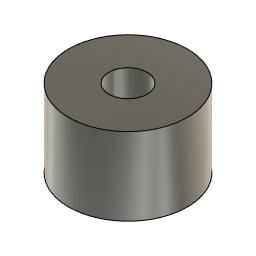
Water_Gun_Stand (Autodesk Fusion 360 archive; units mm, degrees)
design "c-clamp_base_v.1.0.0.0"
Autodesk Fusion 360 part; units mm, degrees
sketch "Base" plane through (0, 0, 0) normal (0, 0, 1) x (1, 0, 0)
  circle A0 centre (0, 0) radius 13
  circle A1 centre (24.2, 0) radius 11.2
  line L0 (25.0331, 11.169) -> (0.9669, 12.964)
  line L1 (0.9669, -12.964) -> (25.0331, -11.169)
  line L2 (0, 0) -> (24.2, 0) construction
  circle A2 centre (24.2, 0) radius 8
  line L3 (9.2469, 9.1375) -> (24.795, 7.9778)
  line L4 (9.2469, -9.1375) -> (24.795, -7.9778)
  line L5 (25.0331, 11.169) -> (24.795, 7.9778)
  line L6 (24.795, -7.9778) -> (25.0331, -11.169)
  dimension "d6" = 16
  dimension "d7" = 3.2
  dimension "d8" = 3.2
  dimension "d9" = 3.2
  dimension "d26" = 26
  constraint coincident A0.centre L2.start
  constraint coincident A1 L0.start
  constraint tangent A1 L0
  constraint coincident A0 L0.end
  constraint tangent A0 L0
  constraint coincident A0 L1.start
  constraint tangent A0 L1
  constraint coincident A1 L1.end
  constraint tangent A1 L1
  constraint coincident A1.centre L2.end
  constraint horizontal L2
  constraint concentric A1 A2
  constraint coincident A0 L3.start
  constraint coincident A2 L3.end
  constraint parallel L0 L3
  constraint coincident A0 L4.start
  constraint coincident A2 L4.end
  constraint parallel L1 L4
  constraint perpendicular L3 L5
  constraint perpendicular L4 L6
  constraint tangent A0 A1
  measures "d6" diameter of A2
  measures "d7" distance of A1 A2
  measures "d8" distance of L1 L4
  measures "d9" distance of L0 L3
  measures "d26" diameter of A0
extrude "Extrude2" add sketch "Base" along normal blind 19 contours A0
sketch "TeeNutInsert" plane through (0, 0, 0) normal (0, 0, 1) x (1, 0, 0)
  circle A0 centre (0, 0) radius 10
  circle A1 centre (0, 0) radius 4.175
  circle A2 centre (0, 0) radius 8.25 construction
  line L0 (6.7415, -0.75) -> (9.7415, -0.75)
  line L1 (9.7415, -0.75) -> (9.7415, 0)
  line L2 (9.7415, 0) -> (6.7415, 0)
  line L3 (6.7415, 0) -> (6.7415, -0.75)
  line L4 (6.7415, -0.75) -> (9.7415, 0) construction
  line L5 (9.7415, -0.75) -> (6.7415, 0) construction
  line L6 (0, 0) -> (8.2415, 0) construction
  point P0 (8.2415, -0.375)
  dimension "d14" = 20
  dimension "d17" = 8.35
  dimension "d18" = 16.5
  dimension "d19" = 3
  dimension "d20" = 0.75
  constraint coincident A0.centre A1.centre
  constraint concentric A0 A1
  constraint concentric A1 A2
  constraint perpendicular L0 L1
  constraint parallel L0 L2
  constraint parallel L1 L3
  constraint horizontal L0
  constraint coincident L4 P0
  constraint coincident L5 P0
  constraint coincident A2 P0
  constraint midpoint L2 L6.end
  constraint horizontal L6
  measures "d14" diameter of A0
  measures "d17" diameter of A1
  measures "d18" diameter of A2
  measures "d19" distance of L1.end L2.end
  measures "d20" distance of L0.end L1.end
extrude "Extrude5" cut sketch "TeeNutInsert" along normal blind 6.5 contours A0 | A1 | L0 L1 L2 L3
extrude "Extrude6" cut sketch "TeeNutInsert" along normal through all contours A1
extrude "Extrude7" cut sketch "TeeNutInsert" along normal blind 10.825 contours L0 L1 L2 L3
pattern_circular "C-Pattern1" count 12 over 360 about axis through (0, 0, 1.75) along (0, 0, 1) of "Extrude7"
chamfer "Chamfer1" distance 0.8 angle 45 1 edges at (-3.8925, -1.5097, 6.5)
sketch "TeeNutSupport" plane through (0, 0, 6.5) normal (0, 0, -1) x (1, 0, 0)
  line L0 (4.8707, 8.4364) -> (3.3707, 5.8383) construction
  line L1 (3.3707, 5.8383) -> (2.7212, 6.2133) construction
  line L2 (2.7212, 6.2133) -> (4.2212, 8.8114) construction
  line L3 (4.2212, 8.8114) -> (4.8707, 8.4364) construction
  line L4 (0, 9.7415) -> (0, 6.7415) construction
  line L5 (0, 6.7415) -> (-0.75, 6.7415) construction
  line L6 (-0.75, 6.7415) -> (-0.75, 9.7415) construction
  line L7 (-0.75, 9.7415) -> (0, 9.7415) construction
  line L8 (-4.8707, 8.4364) -> (-3.3707, 5.8383) construction
  line L9 (-3.3707, 5.8383) -> (-4.0203, 5.4633) construction
  line L10 (-4.0203, 5.4633) -> (-5.5203, 8.0614) construction
  line L11 (-5.5203, 8.0614) -> (-4.8707, 8.4364) construction
  line L12 (-9.7415, 0) -> (-6.7415, 0) construction
  line L13 (-6.7415, 0) -> (-6.7415, -0.75) construction
  line L14 (-6.7415, -0.75) -> (-9.7415, -0.75) construction
  line L15 (-9.7415, -0.75) -> (-9.7415, 0) construction
  line L16 (-4.8707, -8.4364) -> (-3.3707, -5.8383) construction
  line L17 (-3.3707, -5.8383) -> (-2.7212, -6.2133) construction
  line L18 (-2.7212, -6.2133) -> (-4.2212, -8.8114) construction
  line L19 (-4.2212, -8.8114) -> (-4.8707, -8.4364) construction
  line L20 (0, -9.7415) -> (0, -6.7415) construction
  line L21 (0, -6.7415) -> (0.75, -6.7415) construction
  line L22 (0.75, -6.7415) -> (0.75, -9.7415) construction
  line L23 (0.75, -9.7415) -> (0, -9.7415) construction
  line L24 (4.8707, -8.4364) -> (3.3707, -5.8383) construction
  line L25 (3.3707, -5.8383) -> (4.0203, -5.4633) construction
  line L26 (4.0203, -5.4633) -> (5.5203, -8.0614) construction
  line L27 (5.5203, -8.0614) -> (4.8707, -8.4364) construction
  line L28 (9.7415, 0) -> (6.7415, 0) construction
  line L29 (6.7415, 0) -> (6.7415, 0.75) construction
  line L30 (6.7415, 0.75) -> (9.7415, 0.75) construction
  line L31 (9.7415, 0.75) -> (9.7415, 0) construction
  circle A0 centre (0, 0) radius 10
  circle A1 centre (0, 0) radius 4.975
  line L32 (8.4364, -4.8707) -> (5.8383, -3.3707)
  line L33 (5.8383, -3.3707) -> (6.2133, -2.7212)
  line L34 (6.2133, -2.7212) -> (8.8114, -4.2212)
  line L35 (8.8114, -4.2212) -> (8.4364, -4.8707)
  line L36 (-8.4364, -4.8707) -> (-5.8383, -3.3707)
  line L37 (-5.8383, -3.3707) -> (-5.4633, -4.0203)
  line L38 (-5.4633, -4.0203) -> (-8.0614, -5.5203)
  line L39 (-8.0614, -5.5203) -> (-8.4364, -4.8707)
  line L40 (-8.4364, 4.8707) -> (-5.8383, 3.3707)
  line L41 (-5.8383, 3.3707) -> (-6.2133, 2.7212)
  line L42 (-6.2133, 2.7212) -> (-8.8114, 4.2212)
  line L43 (-8.8114, 4.2212) -> (-8.4364, 4.8707)
  line L44 (8.4364, 4.8707) -> (5.8383, 3.3707)
  line L45 (5.8383, 3.3707) -> (5.4633, 4.0203)
  line L46 (5.4633, 4.0203) -> (8.0614, 5.5203)
  line L47 (8.0614, 5.5203) -> (8.4364, 4.8707)
ref_plane "WorkPlane2" through (0, 0, 0.5) normal (0, 0, -1) x (-1, 0, 0)
move_face "OffsetFaces1" offset -2 1 faces at (11.9144, -1.1427, 0)
equation "d4 = 6.5 mm + 12.5 mm"
equation "d22 = 6.5 mm + 4.325 mm"
